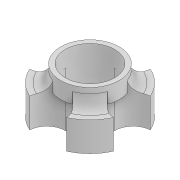
# Autodesk Inventor part: spacer around nuts
Saved by Autodesk Inventor 2020 (Build 240168000, 168)
## iProperties
Created: 2020-02-19
Part Number: spacer around nuts
Material: Generic
Document SubType Name: Modeling
Designer: ball
Density: 1 g/cm^3
Appearance: Default
Author: ball
Autodesk Inventor part; units mm, degrees
ref_plane "YZ Plane" through (0, 0, 0) normal (1, 0, 0) x (0, 1, 0)
ref_plane "XZ Plane" through (0, 0, 0) normal (0, 1, 0) x (-1, 0, 0)
ref_plane "XY Plane" through (0, 0, 0) normal (0, 0, 1) x (1, 0, 0)
sketch "Sketch1" plane through (0, 0, 0) normal (0, 1, 0) x (-1, 0, 0)
  circle A0 centre (9.779, 0) radius 2.8829 construction
  circle A1 centre (-9.779, 0) radius 2.8829 construction
  circle A2 centre (0, 5.9944) radius 2.3114 construction
  circle A3 centre (-5.9944, 0) radius 2.3114 construction
  circle A4 centre (0, -5.9944) radius 2.3114 construction
  circle A5 centre (5.9944, 0) radius 2.3114 construction
  circle A6 centre (0, 0) radius 6.35
  circle A7 centre (0, 5.9944) radius 2.5654
  circle A8 centre (-5.9944, 0) radius 2.5654
  circle A9 centre (0, -5.9944) radius 2.5654
  circle A10 centre (5.9944, 0) radius 2.5654
  dimension "d0" = 5.7658
  dimension "d1" = 5.7658
  dimension "d2" = 9.779
  dimension "d3" = 9.779
  dimension "d4" = 4.6228
  dimension "d5" = 5.9944
  dimension "d8" = 360
  dimension "d10" = 12.7
  dimension "d13" = 5.1308
  dimension "d18" = 360
  constraints: 11 centre point, 4 coincident, 20 other
  measures "d0" diameter of A0
  measures "d1" diameter of A1
  measures "d2" distance of A0.centre point (0, 0)
  measures "d3" distance of A1.centre point (0, 0)
  measures "d4" diameter of A2
  measures "d5" distance of A2.centre point (0, 0)
  measures "d10" diameter of A6
  measures "d13" diameter of A7
extrude "Extrusion1" add sketch "Sketch1" along normal blind 4.064 contours A6 A10 | A10 A6 A9 A8 A7 | A7 A6 | A6 A9 | A8 A6 picked at (5.3827, -0.5032) picked at (0.8457, 5.4356) picked at (0.8457, -5.4356) picked at (-5.4356, -0.8457)
extrude "Extrusion2" cut sketch "Sketch1" along normal through all contours A6 A10 | A6 A10 | A7 A6 | A6 A7 | A9 A6 | A6 A9 | A8 A6 | A6 A8
sketch "Sketch3" plane through (0, 4.064, 0) normal (0, 1, 0) x (1, 0, 0)
  circle A0 centre (0, 0) radius 4.064
  dimension "d20" = 8.128
  constraints: 1 centre point, 1 coincident
  measures "d20" diameter of A0
extrude "Extrusion3" add sketch "Sketch3" along normal blind 2.286
sketch "Sketch4" plane through (0, 6.35, 0) normal (0, 1, 0) x (1, 0, 0)
  circle A0 centre (0, 0) radius 3.429
  dimension "d23" = 6.858
  constraints: 1 centre point, 1 coincident
  measures "d23" diameter of A0
extrude "Extrusion4" cut sketch "Sketch4" against normal through all
fillet "Fillet1" radius 1.524 4 edges at (2.8737, 4.064, -2.8737) (2.8737, 4.064, 2.8737) (-2.8737, 4.064, -2.8737) (-2.8737, 4.064, 2.8737)
equation "\"d1\" = d0"
equation "\"d3\" = d2"
body "Solid1"
